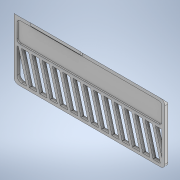
# Autodesk Inventor part: top rev5 part2
Saved by Autodesk Inventor 2021 (Build 250183000, 183)
## iProperties
Created: 2024-09-23
Part Number: top rev5 part2
Material: Generic
Document SubType Name: Modeling
Designer: Toby
Density: 1 g/cm^3
Appearance: Default
Author: Toby
Autodesk Inventor part; units mm, degrees
ref_plane "YZ Plane" through (0, 0, 0) normal (1, 0, 0) x (0, 1, 0)
ref_plane "XZ Plane" through (0, 0, 0) normal (0, 1, 0) x (-1, 0, 0)
ref_plane "XY Plane" through (0, 0, 0) normal (0, 0, 1) x (1, 0, 0)
sketch "Sketch1" plane through (0, 0, 0) normal (0, 0, 1) x (1, 0, 0)
  line L0 (-50, 19.75) -> (50, 19.75)
  line L1 (50, 19.75) -> (50, -19.75)
  line L2 (50, -19.75) -> (-50, -19.75)
  line L3 (-50, -19.75) -> (-50, 19.75)
  line L4 (-48, 17.75) -> (48, 17.75)
  line L5 (48, 17.75) -> (48, -17.75)
  line L6 (48, -17.75) -> (-48, -17.75)
  line L7 (-48, -17.75) -> (-48, 17.75)
  point P0 (0, 0)
  dimension "d0" = 39.5
  dimension "d1" = 100
  dimension "d2" = 19.75
  dimension "d3" = 50
  dimension "d4" = 2
  dimension "d5" = 2
  dimension "d6" = 2
  dimension "d7" = 2
  constraints: 16 end point, 4 parallel, 2 horizontal, 2 perpendicular
  measures "d0" distance of L2.end L0.start
  measures "d1" distance of L0.start L0.end
  measures "d2" distance from line of point (0, 0) L0
  measures "d3" distance from line of point (0, 0) L3
  measures "d4" distance between parallel lines of L4 L0
  measures "d5" distance between parallel lines of L2 L6
  measures "d6" distance between parallel lines of L3 L7
  measures "d7" distance between parallel lines of L1 L5
extrude "Extrusion1" add sketch "Sketch1" along normal blind 2
sketch "Sketch2" plane through (0, 0, 0) normal (0, 0, -1) x (-1, 0, 0)
  line L0 (-48, -17.75) -> (-38.4878, 17.75) construction
  line L1 (48, 17.75) -> (-48, 17.75) projected
  line L2 (-47.0341, -18.0088) -> (-37.5219, 17.4912)
  line L3 (-39.4537, 18.0088) -> (-48.9659, -17.4912)
  arc A0 (-48.9659, -17.4912) -> (-47.0341, -18.0088) centre (-48, -17.75) ccw
  arc A1 (-37.5219, 17.4912) -> (-39.4537, 18.0088) centre (-38.4878, 17.75) ccw
  line L4 (-48, -17.75) -> (-11.2477, -17.75) construction
  line L5 (-48, -17.75) -> (48, -17.75) projected
  line L6 (-41.1758, -17.75) -> (-31.5943, 18.0088) construction
  line L7 (-40.2099, -18.0088) -> (-30.6284, 17.75)
  line L8 (-32.5602, 18.2676) -> (-42.1418, -17.4912)
  arc A2 (-42.1418, -17.4912) -> (-40.2099, -18.0088) centre (-41.1758, -17.75) ccw
  arc A3 (-30.6284, 17.75) -> (-32.5602, 18.2676) centre (-31.5943, 18.0088) ccw
  line L9 (-33.3857, -18.0088) -> (-23.8042, 17.75)
  line L10 (-25.736, 18.2676) -> (-35.3176, -17.4912)
  arc A4 (-35.3176, -17.4912) -> (-33.3857, -18.0088) centre (-34.3517, -17.75) ccw
  arc A5 (-23.8042, 17.75) -> (-25.736, 18.2676) centre (-24.7701, 18.0088) ccw
  line L11 (-26.5616, -18.0088) -> (-16.98, 17.75)
  line L12 (-18.9119, 18.2676) -> (-28.4934, -17.4912)
  arc A6 (-28.4934, -17.4912) -> (-26.5616, -18.0088) centre (-27.5275, -17.75) ccw
  arc A7 (-16.98, 17.75) -> (-18.9119, 18.2676) centre (-17.9459, 18.0088) ccw
  line L13 (-19.7374, -18.0088) -> (-10.1558, 17.75)
  line L14 (-12.0877, 18.2676) -> (-21.6692, -17.4912)
  arc A8 (-21.6692, -17.4912) -> (-19.7374, -18.0088) centre (-20.7033, -17.75) ccw
  arc A9 (-10.1558, 17.75) -> (-12.0877, 18.2676) centre (-11.1218, 18.0088) ccw
  line L15 (-12.9132, -18.0088) -> (-3.3317, 17.75)
  line L16 (-5.2635, 18.2676) -> (-14.8451, -17.4912)
  arc A10 (-14.8451, -17.4912) -> (-12.9132, -18.0088) centre (-13.8791, -17.75) ccw
  arc A11 (-3.3317, 17.75) -> (-5.2635, 18.2676) centre (-4.2976, 18.0088) ccw
  line L17 (-6.089, -18.0088) -> (3.4925, 17.75)
  line L18 (1.5607, 18.2676) -> (-8.0209, -17.4912)
  arc A12 (-8.0209, -17.4912) -> (-6.089, -18.0088) centre (-7.055, -17.75) ccw
  arc A13 (3.4925, 17.75) -> (1.5607, 18.2676) centre (2.5266, 18.0088) ccw
  line L19 (0.7351, -18.0088) -> (10.3167, 17.75)
  line L20 (8.3848, 18.2676) -> (-1.1967, -17.4912)
  arc A14 (-1.1967, -17.4912) -> (0.7351, -18.0088) centre (-0.2308, -17.75) ccw
  arc A15 (10.3167, 17.75) -> (8.3848, 18.2676) centre (9.3508, 18.0088) ccw
  line L21 (7.5593, -18.0088) -> (17.1409, 17.75)
  line L22 (15.209, 18.2676) -> (5.6275, -17.4912)
  arc A16 (5.6275, -17.4912) -> (7.5593, -18.0088) centre (6.5934, -17.75) ccw
  arc A17 (17.1409, 17.75) -> (15.209, 18.2676) centre (16.1749, 18.0088) ccw
  line L23 (14.3835, -18.0088) -> (23.965, 17.75)
  line L24 (22.0332, 18.2676) -> (12.4516, -17.4912)
  arc A18 (12.4516, -17.4912) -> (14.3835, -18.0088) centre (13.4176, -17.75) ccw
  arc A19 (23.965, 17.75) -> (22.0332, 18.2676) centre (22.9991, 18.0088) ccw
  line L25 (21.2077, -18.0088) -> (30.7892, 17.75)
  line L26 (28.8573, 18.2676) -> (19.2758, -17.4912)
  arc A20 (19.2758, -17.4912) -> (21.2077, -18.0088) centre (20.2417, -17.75) ccw
  arc A21 (30.7892, 17.75) -> (28.8573, 18.2676) centre (29.8233, 18.0088) ccw
  line L27 (28.0318, -18.0088) -> (37.6134, 17.75)
  line L28 (35.6815, 18.2676) -> (26.1, -17.4912)
  arc A22 (26.1, -17.4912) -> (28.0318, -18.0088) centre (27.0659, -17.75) ccw
  arc A23 (37.6134, 17.75) -> (35.6815, 18.2676) centre (36.6474, 18.0088) ccw
  line L29 (34.856, -18.0088) -> (44.4375, 17.75)
  line L30 (42.5057, 18.2676) -> (32.9241, -17.4912)
  arc A24 (32.9241, -17.4912) -> (34.856, -18.0088) centre (33.8901, -17.75) ccw
  arc A25 (44.4375, 17.75) -> (42.5057, 18.2676) centre (43.4716, 18.0088) ccw
  line L31 (41.6802, -18.0088) -> (51.2617, 17.75)
  line L32 (49.3299, 18.2676) -> (39.7483, -17.4912)
  arc A26 (39.7483, -17.4912) -> (41.6802, -18.0088) centre (40.7142, -17.75) ccw
  arc A27 (51.2617, 17.75) -> (49.3299, 18.2676) centre (50.2958, 18.0088) ccw
  line L33 (-53.9276, -18.0088) -> (-44.4154, 17.4912)
  line L34 (-46.3473, 18.0088) -> (-55.8594, -17.4912)
  arc A28 (-55.8594, -17.4912) -> (-53.9276, -18.0088) centre (-54.8935, -17.75) ccw
  arc A29 (-44.4154, 17.4912) -> (-46.3473, 18.0088) centre (-45.3813, 17.75) ccw
  point P0 (0, 0)
  point P1 (45, 17.75)
  point P2 (-45, 17.75)
  point P3 (-43.2439, 0)
  point P4 (-45, -17.75)
  point P5 (45, -17.75)
  point P6 (-36.3851, 0.1294)
  point P7 (32.8901, -17.75)
  point P8 (34.9253, -17.75)
  point P9 (42.367, 17.75)
  point P10 (26.0659, -17.75)
  point P11 (28.1012, -17.75)
  point P12 (35.5428, 17.75)
  point P13 (5.5934, -17.75)
  point P14 (7.6287, -17.75)
  point P15 (15.0703, 17.75)
  point P16 (-1.2308, -17.75)
  point P17 (0.8045, -17.75)
  point P18 (8.2461, 17.75)
  point P19 (-8.055, -17.75)
  point P20 (-6.0197, -17.75)
  point P21 (1.422, 17.75)
  point P22 (-42.1758, -17.75)
  point P23 (-40.1406, -17.75)
  point P24 (-32.6989, 17.75)
  point P25 (-37.4878, 17.75)
  point P26 (-39.5231, 17.75)
  dimension "d11" = 75
  dimension "d12" = 2
  dimension "d13" = 2
  dimension "d14" = 2
  dimension "d15" = 2
  dimension "d16" = 2
  dimension "d17" = 2
  dimension "d18" = 2
  dimension "d19" = 2
  dimension "d20" = 2
  dimension "d21" = 2
  dimension "d22" = 2
  dimension "d23" = 2
  dimension "d24" = 2
  dimension "d25" = 2
  dimension "d26" = 2
  constraints: 70 end point, 60 point on circle, 60 tangent, 30 centre point, 16 parallel, 2 midpoint, 2 point on line, 1 equal length, 1 horizontal
  measures "d11" angle of L4 L0
  measures "d12" diameter of A1
  measures "d13" diameter of A3
  measures "d14" diameter of A5
  measures "d15" diameter of A7
  measures "d16" diameter of A9
  measures "d17" diameter of A11
  measures "d18" diameter of A13
  measures "d19" diameter of A15
  measures "d20" diameter of A17
  measures "d21" diameter of A19
  measures "d22" diameter of A21
  measures "d23" diameter of A23
  measures "d24" diameter of A25
  measures "d25" diameter of A27
  measures "d26" diameter of A29
extrude "Extrusion2" add sketch "Sketch2" against normal blind 2 contours L29 L5 A24 L30 L1 | L27 L5 A22 L28 L1 | L25 L5 A20 L26 L1 | L1 L26 A21 | L25 A20 L5 | L23 L5 A18 L24 L1 | L1 L24 A19 | L23 A18 L5 | L21 L5 A16 L22 L1 | L19 L5 A14 L20 L1 | L17 L5 A12 L18 L1 | L15 L5 A10 L16 L1 | L1 L16 A11 | L15 A10 L5 | L13 L5 A8 L14 L1 | L1 L14 A9 | L13 A8 L5 | L11 L5 A6 L12 L1 | L1 L12 A7 | L11 A6 L5 | L9 L5 A4 L10 L1 | L1 L10 A5 | L9 A4 L5 | L7 L5 A2 L8 L1 | A1 L2 A0 L3 L1
sketch "Sketch3" plane through (0, 0, 0) normal (0, 0, -1) x (-1, 0, 0)
  line L0 (34.9253, -17.75) -> (48, -17.75) projected
  line L1 (40.7146, -17.75) -> (48, 9.4394) construction
  line L2 (48, -17.75) -> (48, 17.75) projected
  line L3 (41.6805, -18.0088) -> (48.9659, 9.1806)
  line L4 (47.0341, 9.6983) -> (39.7487, -17.4912)
  arc A0 (39.7487, -17.4912) -> (41.6805, -18.0088) centre (40.7146, -17.75) ccw
  arc A1 (48.9659, 9.1806) -> (47.0341, 9.6983) centre (48, 9.4394) ccw
  line L5 (34.9253, -17.75) -> (44.4375, 17.75) projected
  line L6 (28.1012, -17.75) -> (37.6134, 17.75) projected
  line L7 (42.367, 17.75) -> (32.9241, -17.4912) projected
  point P0 (0, 0)
  point P1 (45, -17.75)
  point P2 (48, -14.75)
  point P3 (48, 14.75)
  point P4 (44.3573, -4.1553)
  point P5 (39.7146, -17.75)
  point P6 (41.7499, -17.75)
  point P7 (48, 5.5757)
  point P8 (48, 10.4394)
  dimension "d33" = 2
  dimension "d34" = 4.5916
  dimension "d35" = 5.592
  constraints: 8 end point, 4 point on circle, 4 tangent, 2 centre point, 2 parallel, 2 point on line, 1 midpoint
  measures "d33" diameter of A1
  measures "d34" distance between parallel lines of L6 L7
  measures "d35" distance between parallel lines of L5 L1
extrude "Extrusion3" add sketch "Sketch3" against normal blind 2 contours A0 L4 A1 L2 L3 L0
sketch "Sketch5" plane through (0, 0, 0) normal (0, 0, -1) x (-1, 0, 0)
  line L0 (48, 5.5757) -> (41.7499, -17.75) projected
  line L1 (48, 5.5757) -> (46.0681, 6.0934)
  line L2 (46.0681, 6.0934) -> (48, 13.3031)
  line L3 (48, 13.3031) -> (48, 5.5757)
  line L4 (47.0341, 9.6983) -> (39.7487, -17.4912) projected
  line L5 (48, 10.4394) -> (48, 5.5757) projected
  point P0 (0, 0)
  point P1 (48, 14.75)
  constraints: 6 end point, 2 collinear, 2 perpendicular
extrude "Extrusion5" add sketch "Sketch5" against normal blind 2
sketch "Sketch6" plane through (-50, -19.75, 0) normal (-1, 0, 0) x (0, 0, 1)
  line L0 (0, 39.5) -> (2, 39.5) projected
  line L1 (2, 39.5) -> (0, 37.2074)
  line L2 (0, 39.5) -> (0, 0) projected
  line L3 (0, 37.2074) -> (0, 39.5)
  line L4 (0, 39.5) -> (2, 39.5)
  point P0 (0, 19.75)
  constraints: 6 end point, 1 perpendicular, 1 point on line, 1 vertical
extrude "Extrusion6" cut sketch "Sketch6" against normal blind 300
fillet "Fillet3" radius 3 3 edges at (-50, -19.75, 1) (50, -19.75, 1) (-48, -17.75, 1)
sketch "Sketch7" plane through (0, 0, 0) normal (0, 0, -1) x (-1, 0, 0)
  line L0 (-50, -16.75) -> (-50, 17.4574) projected
  line L1 (-50, 19.75) -> (50, 19.75) projected
  line L2 (-50, 17.4574) -> (-50, 19.75) projected
  circle A0 centre (-47, 16.75) radius 3
  line L3 (-50, 16.75) -> (-47, 16.75)
  line L4 (-47, 16.75) -> (-47, 19.75)
  line L5 (-47, 19.75) -> (-50, 19.75)
  line L6 (-50, 19.75) -> (-50, 16.75)
  point P0 (0, 0)
  dimension "d46" = 3
  dimension "d47" = 3
  constraints: 8 end point, 3 point on line, 2 parallel, 2 point on circle, 1 centre point, 1 coincident, 1 horizontal, 1 perpendicular
  measures "d46" distance of L1.start L3.start
  measures "d47" distance of point (-47, 19.75) L1.start
extrude "Extrusion7" cut sketch "Sketch7" against normal blind 300 contours L0 L2 L1 A0
fillet "Fillet4" radius 3 1 edges at (48, 17.75, 1.1276)
sketch "Sketch8" plane through (0, 0, 0) normal (0, 0, -1) x (-1, 0, 0)
  line L0 (48, 13.3031) -> (48, 17.4574) projected
  line L1 (-48, 14.75) -> (-48, -13.8863) projected
  line L2 (48, 17.4574) -> (-48, 17.4574)
  line L3 (-48, 17.4574) -> (-48, 2.25)
  line L4 (-48, 2.25) -> (48, 2.25)
  line L5 (48, 2.25) -> (48, 17.4574)
  line L6 (14.4528, -17.75) -> (19.2417, -17.75) projected
  point P0 (0, 0)
  dimension "d51" = 20
  constraints: 8 end point, 2 parallel, 1 horizontal, 1 perpendicular, 1 point on line
  measures "d51" distance between parallel lines of L4 L6
extrude "Extrusion8" add sketch "Sketch8" against normal blind 2
sketch "Sketch9" plane through (-50, -16.75, 0) normal (-1, 0, 0) x (0, 0, 1)
  line L0 (2, 33.5) -> (0, 33.5) projected
  line L1 (0, 34.2074) -> (0, 0) projected
  line L2 (0, 33.5) -> (0, 34.2074)
  line L3 (2, 36.5) -> (0, 34.2074) projected
  line L4 (0, 34.2074) -> (2, 36.5)
  line L5 (2, 0) -> (2, 33.5) projected
  line L6 (2, 36.5) -> (2, 33.5)
  line L7 (2, 33.5) -> (0, 33.5)
  point P0 (0, 16.75)
  constraints: 8 end point, 1 collinear, 1 parallel, 1 perpendicular, 1 vertical
extrude "Extrusion9" add sketch "Sketch9" against normal blind 97
sketch "Sketch11" plane through (49.9154, 17.4574, 0) normal (0, 0.6573904, -0.7535502) x (-1, 0, 0)
  line L0 (2.9154, 3.0423) -> (99.9154, 3.0423) projected
  line L1 (87.8154, 3.0423) -> (54.8154, 3.0423)
  line L2 (54.8154, 3.0423) -> (54.8154, 4.8423)
  line L3 (54.8154, 4.8423) -> (87.8154, 4.8423)
  line L4 (87.8154, 4.8423) -> (87.8154, 3.0423)
  line L5 (99.9154, 3.0423) -> (99.9154, 0) projected
  line L6 (87.8154, 3.0423) -> (54.8154, 3.0423)
  line L7 (54.8154, 3.0423) -> (54.8154, 1.0423)
  line L8 (54.8154, 1.0423) -> (87.8154, 1.0423)
  line L9 (87.8154, 1.0423) -> (87.8154, 3.0423)
  point P0 (49.9154, -13.1551)
  point P1 (54.8154, 3.0423)
  point P2 (54.8154, 3.0423)
  point P3 (54.8154, 3.0423)
  point P4 (54.8154, 3.0423)
  dimension "d62" = 12.1
  dimension "d63" = 33
  dimension "d64" = 1.8
  dimension "d65" = 2
  constraints: 16 end point, 4 parallel, 2 horizontal, 2 perpendicular, 1 point on line
  measures "d62" distance between parallel lines of L5 L4
  measures "d63" distance of L2.end L3.end
  measures "d64" distance between parallel lines of L0 L3
  measures "d65" distance of L7.end L6.end
extrude "Extrusion11" add sketch "Sketch11" against normal blind 1.2
chamfer "Chamfer2" distance 1.2 angle 45 1 edges at (-21.4, 20.3175, 4.0876)
sketch "Sketch12" plane through (0, 0, 2) normal (0, 0, 1) x (1, 0, 0)
  line L0 (-48, 4.25) -> (48, 4.25)
  line L1 (48, 4.25) -> (48, 17.75)
  line L2 (48, 17.75) -> (-48, 17.75)
  line L3 (-48, 17.75) -> (-48, 4.25)
  line L4 (-50, 19.75) -> (-50, -16.75) projected
  line L5 (50, -16.75) -> (50, 16.75) projected
  line L6 (-4.0929, 2.25) -> (0.6607, 2.25) projected
  line L7 (47, 19.75) -> (-4.9, 19.75) projected
  point P0 (0, 0)
  dimension "d71" = 2
  dimension "d72" = 2
  dimension "d73" = 2
  dimension "d74" = 2
  constraints: 8 end point, 2 parallel, 1 horizontal, 1 perpendicular
  measures "d71" distance between parallel lines of L3 L4
  measures "d72" distance between parallel lines of L5 L1
  measures "d73" distance between parallel lines of L6 L0
  measures "d74" distance between parallel lines of L7 L2
extrude "Extrusion12" cut sketch "Sketch12" against normal blind 0.8
fillet "Fillet5" radius 2 4 edges at (-48, 4.25, 1.6) (-48, 17.75, 1.6) (48, 4.25, 1.6) (48, 17.75, 1.6)
body "Solid1"
